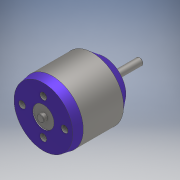
# Autodesk Inventor part: Brushless Motor
Saved by Autodesk Inventor 2017 (Build 210142000, 142)
## iProperties
Created: 2017-08-01
Part Number: Brushless Motor
Material: Generic
Document SubType Name: Modeling
Designer: Thein Lin Aung
Density: 1 g/cm^3
Appearance: Default
Author: Thein Lin Aung
Autodesk Inventor part; units mm, degrees
ref_plane "YZ Plane" through (0, 0, 0) normal (1, 0, 0) x (0, 1, 0)
ref_plane "XZ Plane" through (0, 0, 0) normal (0, 1, 0) x (-1, 0, 0)
ref_plane "XY Plane" through (0, 0, 0) normal (0, 0, 1) x (1, 0, 0)
sketch "Sketch1" plane through (0, 0, 0) normal (0, 1, 0) x (-1, 0, 0)
  circle A0 centre (0, 0) radius 13.85
  dimension "d0" = 27.7
  constraints: 1 centre point, 1 coincident
  measures "d0" diameter of A0
extrude "Extrusion1" add sketch "Sketch1" along normal blind 22
sketch "Sketch2" plane through (0, 0, 0) normal (1, 0, 0) x (0, 1, 0)
  line L0 (22, -13.85) -> (22, 13.85) projected
  line L1 (-4.4, 0) -> (26.4, 0) projected
  line L2 (22, -13.85) -> (27.25, -9.65)
  line L3 (27.25, -9.65) -> (27.25, 0)
  line L4 (22, 0) -> (22, -13.85)
  line L5 (27.25, 0) -> (22, 0)
  point P0 (0, 0)
  dimension "d3" = 5.25
  dimension "d6" = 9.65
  constraints: 8 end point, 2 perpendicular, 2 point on line, 1 collinear, 1 midpoint
  measures "d3" distance between parallel lines of L0 L3
  measures "d6" distance of L2.end L3.end
revolve "Revolution1" add sketch "Sketch2" angle 360 about axis through (0, -10, 0) along (0, 1, 0)
chamfer "Chamfer1" distance 4 angle 10 1 edges at (13.85, 0, 0) measured on face at (13.85, 0.5, 0)
sketch "Sketch3" plane through (0, 27.25, 0) normal (0, 1, 0) x (1, 0, 0)
  circle A0 centre (0, 0) radius 1.58
  dimension "d10" = 3.16
  constraints: 1 centre point, 1 coincident
  measures "d10" diameter of A0
extrude "Extrusion2" add sketch "Sketch3" along normal blind 15.82
sketch "Sketch4" plane through (0, 27.25, 0) normal (0, 1, 0) x (1, 0, 0)
  circle A0 centre (0, 0) radius 4.485
  dimension "d13" = 8.97
  constraints: 1 centre point, 1 coincident
  measures "d13" diameter of A0
extrude "Extrusion3" add sketch "Sketch4" along normal blind 2
sketch "Sketch5" plane through (0, 27.25, 0) normal (0, 1, 0) x (1, 0, 0)
  line L0 (0, 19.39) -> (0, -19.39) projected
  circle A0 centre (0, 6) radius 1
  point P0 (0, 0)
  dimension "d16" = 6
  dimension "d17" = 2
  constraints: 1 centre point, 1 point on line
  measures "d16" distance of point (0, 0) A0.centre
  measures "d17" diameter of A0
extrude "Extrusion4" cut sketch "Sketch5" against normal blind 3
thread "Thread1" size "M2x0.4" class "6H" standard "ANSI Metric M Profile" full length
pattern_circular "Circular Pattern1" count 4 over 360 about axis through (0, -10, 0) along (0, 1, 0) of "Extrusion4"
sketch "Sketch6" plane through (0, 0, 0) normal (0, -1, 0) x (1, 0, 0)
  line L0 (-19.39, 0) -> (19.39, 0) projected
  line L1 (0, -19.39) -> (0, 19.39) projected
  circle A0 centre (9.5, 0) radius 1.5
  circle A1 centre (0, 8) radius 1.5
  circle A2 centre (-9.5, 0) radius 1.5
  circle A3 centre (0, -8) radius 1.5
  point P0 (0, 0)
  dimension "d25" = 9.5
  dimension "d26" = 8
  dimension "d27" = 3
  constraints: 4 centre point, 2 point on line, 2 symmetric about line, 1 equal radius, 2 other
  measures "d25" distance from line of L1 A0.centre
  measures "d26" distance from line of A1.centre L0
  measures "d27" diameter of A0
extrude "Extrusion5" cut sketch "Sketch6" against normal blind 5
thread "Thread2" size "M3x0.5" class "6H" standard "ANSI Metric M Profile" full length
thread "Thread3" size "M3x0.5" class "6H" standard "ANSI Metric M Profile" full length
thread "Thread4" size "M3x0.5" class "6H" standard "ANSI Metric M Profile" full length
thread "Thread5" size "M3x0.5" class "6H" standard "ANSI Metric M Profile" full length
sketch "Sketch7" plane through (0, 0, 0) normal (0, -1, 0) x (1, 0, 0)
  circle A0 centre (0, 0) radius 4.75
  dimension "d38" = 9.5
  constraints: 1 centre point, 1 coincident
  measures "d38" diameter of A0
extrude "Extrusion6" cut sketch "Sketch7" against normal blind 0.3
sketch "Sketch8" plane through (0, 0.3, 0) normal (0, -1, 0) x (1, 0, 0)
  circle A0 centre (0, 0) radius 1.58 projected
extrude "Extrusion7" add sketch "Sketch8" along normal blind 1.7
chamfer "Chamfer2" distance 0.2 angle 45 2 edges at (-1.58, -1.4, 0) (-1.58, 43.07, 0)
body "Solid1"
